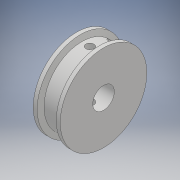
# Autodesk Inventor part: spool v2
Saved by Autodesk Inventor 2017 (Build 210142000, 142)
## iProperties
Created: 2018-07-31
Part Number: spool v2
Material: Generic
Document SubType Name: Modeling
Designer: jakub.tomczynski
Density: 1 g/cm^3
Appearance: Default
Author: jakub.tomczynski
## iProperties of the stored document spool v2_3DPrint.ipt
Created: 2018-08-31
Part Number: spool v2_3DPrint
Material: Generic
Document SubType Name: Modeling
Designer: jakub.tomczynski
Density: 1 g/cm^3
Appearance: Default
Author: jakub.tomczynski
Autodesk Inventor part; units mm, degrees
ref_plane "YZ Plane" through (0, 0, 0) normal (1, 0, 0) x (0, 1, 0)
ref_plane "XZ Plane" through (0, 0, 0) normal (0, 1, 0) x (-1, 0, 0)
ref_plane "XY Plane" through (0, 0, 0) normal (0, 0, 1) x (1, 0, 0)
sketch "Sketch1" plane through (0, 0, 0) normal (0, 0, 1) x (1, 0, 0)
  line L0 (-2.5, 0) -> (-2.5, 8)
  line L1 (-2.5, 8) -> (-1.7679, 8)
  line L2 (-1.7679, 8) -> (-1.5, 7)
  line L3 (-1.5, 7) -> (0, 7)
  line L4 (0, 0) -> (0, 14.5205) construction
  line L5 (-2.5, 0) -> (2.5, 0)
  line L6 (2.5, 0) -> (2.5, 8)
  line L7 (2.5, 8) -> (1.7679, 8)
  line L8 (1.7679, 8) -> (1.5, 7)
  line L9 (1.5, 7) -> (0, 7)
  dimension "d0" = 5
  dimension "d1" = 16
  dimension "d2" = 14
  dimension "d3" = 3
  dimension "d4" = 15
  constraints: 20 end point, 4 symmetric about line, 2 vertical, 1 horizontal, 1 midpoint, 1 parallel, 1 perpendicular
  measures "d0" distance between parallel lines of L6 L0
  measures "d1" diameter of L7 L5
  measures "d2" diameter of L9 L5
  measures "d3" distance of L9.start L2.end
  measures "d4" angle of L4 L8
revolve "Revolution1" add sketch "Sketch1" angle 360 about axis through (-2.5, 0, 0) along (1, 0, 0)
sketch "Sketch2" plane through (0, 0, 0) normal (0, 0, 1) x (1, 0, 0)
  circle A0 centre (0, 0) radius 0.75
  dimension "d6" = 1.5
  constraints: 1 centre point, 1 coincident
  measures "d6" diameter of A0
extrude "Extrusion1" cut sketch "Sketch2" along normal blind 10 and the other way blind 10
sketch "Sketch4" plane through (-2.5, 0, 0) normal (-1, 0, 0) x (0, 0, 1)
  circle A0 centre (0, 0) radius 2
  dimension "d18" = 4
  constraints: 1 centre point, 1 coincident
  measures "d18" diameter of A0
extrude "Extrusion2" cut sketch "Sketch4" against normal through all
sketch "Sketch7" plane through (0, 0, 0) normal (0, 0, 1) x (1, 0, 0)
  circle A0 centre (0, 4.5) radius 1
  point P0 (0, 0)
  dimension "d32" = 2
  dimension "d33" = 4.5
  constraints: 1 centre point, 1 vertical alignment
  measures "d32" diameter of A0
  measures "d33" distance of A0.centre point (0, 0)
extrude "Extrusion3" cut sketch "Sketch7" along normal through all both and the other way through all
body "Solid1"
